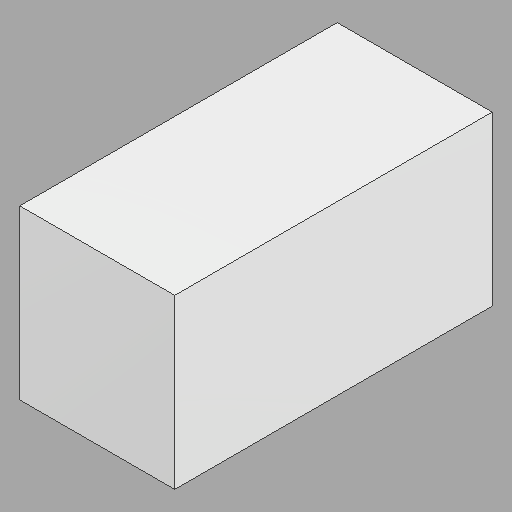
# Autodesk Inventor part: BATTERY
Saved by Autodesk Inventor 2025.2 (Build 292293000, 293)
## iProperties
Created: 2026-09-02
Part Number: BATTERY
Material: ABS Plastic
Document SubType Name: Modeling
Designer: Ben
Mass: 2721.55 g
Surface Area: 737.6 cm^2
Volume: 1269.9 cm^3
Density: 2.14312 g/cm^3
Appearance: Smooth - White
Author: Ben
Autodesk Inventor part; units mm, degrees
ref_plane "YZ Plane" through (0, 0, 0) normal (1, 0, 0) x (0, 1, 0)
ref_plane "XZ Plane" through (0, 0, 0) normal (0, 1, 0) x (-1, 0, 0)
ref_plane "XY Plane" through (0, 0, 0) normal (0, 0, 1) x (1, 0, 0)
sketch "Sketch1" plane through (0, 0, 0) normal (0, 0, 1) x (1, 0, 0)
  line L0 (-41.5, -45) -> (41.5, -45)
  line L1 (41.5, -45) -> (41.5, 45)
  line L2 (41.5, 45) -> (-41.5, 45)
  line L3 (-41.5, 45) -> (-41.5, -45)
  line L4 (-41.5, -45) -> (41.5, 45) construction
  line L5 (41.5, -45) -> (-41.5, 45) construction
  point P0 (0, 0)
  dimension "d0" = 90
  dimension "d1" = 83
  constraints: 12 end point, 2 midpoint, 2 parallel, 1 horizontal, 1 perpendicular
  measures "d0" distance of L0.end L1.end
  measures "d1" distance of L1.end L2.end
extrude "Extrusion1" add sketch "Sketch1" along normal blind 170
body "Solid1"
